13cmholder2 (Autodesk Fusion 360 design; units mm, degrees)
Autodesk Fusion 360 part; units mm, degrees
note: some values were not read from the file. Chosen so that the rebuilt part matches the saved one: that a step has no effect; which face or edge a step refers to. Set by a fixed rule: which sketch regions a step uses.
sketch "Sketch1" plane through (0, 0, 0) normal (1, 0, 0) x (0, 1, 0)
  line L0 (13, -20) -> (-13, 20) construction
  line L1 (-13, -20) -> (13, 20) construction
  line L2 (21.7, -15.8) -> (-8.7, -15.8)
  line L3 (21.7, 15.8) -> (25.9, 15.8)
  line L4 (6.5, -15.8) -> (-34.8, -15.8)
  line L5 (8.6, -15.8) -> (50, -15.8)
  line L6 (50, -15.8) -> (50, -24.8)
  line L7 (50, -24.8) -> (0, -24.8)
  line L8 (-31.55, -27.4) -> (-31.55, 4.2)
  line L9 (-35.75, -15.8) -> (-35.75, 4.2)
  line L10 (-31.55, 4.2) -> (-35.75, 4.2)
  line L11 (-23.95, -27.4) -> (-23.95, 4.2)
  line L12 (-19.75, -27.4) -> (-19.75, 4.2)
  line L13 (-19.75, 4.2) -> (-23.95, 4.2)
  line L14 (-34.8, -15.8) -> (-35.75, -15.8)
  line L15 (-34.8, -20) -> (-35.75, -20)
  line L16 (-35, -24.8) -> (-9, -24.8)
  line L17 (-9, -24.8) -> (0, -24.8)
  line L18 (-35.75, -15.8) -> (-35.75, -24.8)
  line L19 (-35, -24.8) -> (-35.75, -24.8)
  line L20 (-19.75, 4.2) -> (-19.75, 36.6079)
  line L21 (0.25, -15.8) -> (0.25, 36.6079)
  line L22 (-19.75, 36.6079) -> (0.25, 36.6079)
  line L23 (-22.9842, 4.2) -> (-17.5458, 4.2)
  line L24 (-17.5458, 4.2) -> (-17.5458, 36.6079)
  line L25 (-22.6003, 36.6079) -> (-22.9842, 4.2)
  line L26 (-17.5458, 36.6079) -> (-22.6003, 36.6079)
  dimension "d49" = 4.2
  dimension "d50" = 7.6
  dimension "d51" = 4.2
  dimension "d59" = 9
  dimension "d81" = 20
  dimension "d82" = 20
  dimension "d84" = 20
  constraint coincident L0 origin
  constraint coincident L1 origin
  constraint horizontal L4
  constraint midpoint L2 L4.start
  constraint perpendicular L8 L10
  constraint perpendicular L12 L13
  constraint perpendicular L9 L14
  constraint parallel L7 L17
  constraint perpendicular L15 L18
  constraint perpendicular L18 L19
  constraint perpendicular L13 L20
  constraint coincident L4 L21.start
  constraint perpendicular L4 L21
  constraint perpendicular L21 L22
  constraint coincident L13 L23.start
  constraint perpendicular L20 L23
  constraint coincident L22 L24.end
  constraint perpendicular L22 L24
  constraint parallel L22 L26
  measures "d49" distance of L9.end L8.end
  measures "d50" distance of L8 L11
  measures "d51" distance of L11 L12
  measures "d59" distance of L5 L7
  measures "d81" distance of L4 L10
  measures "d82" distance of L4 L13
  measures "d84" distance of L20 L21
extrude "Extrude1" add sketch "Sketch1" along normal mid plane 90 contours L2 L4 L5 L6 L7 L12 L16 L17 | L4 L11 L12 L16 | L4 L8 L11 L16 | L4 L8 L14 L16 L18 L19
extrude "Extrude5" [no effect]
extrude "Extrude6" add sketch "Sketch1" along normal mid plane 90 contours L4 L11 L12 L13 L23 | L4 L8 L9 L10 L14
sketch "Sketch6" plane through (0, -35.75, 0) normal (0, -1, 0) x (1, 0, 0)
  line L0 (-45, -24.8) -> (45, -24.8)
  line L1 (45, -24.8) -> (45, 4.2)
  line L2 (45, 4.2) -> (-45, 4.2)
  line L3 (-45, 4.2) -> (-45, -24.8)
  line L4 (0, 4.2) -> (0, -1.8)
  line L5 (0, -1.8) -> (28.1, -1.8)
  circle A0 centre (28.1, -1.8) radius 3
  line L6 (0, -15.8) -> (0, 4.2)
  circle A1 centre (-28.1, -1.8) radius 3
  line L7 (-24.7214, -20.3) -> (-24.7214, -10.3)
  line L8 (-24.7214, -10.3) -> (-23.398, -10.3)
  line L9 (-23.398, -10.3) -> (-23.398, -20.3)
  line L10 (-23.398, -20.3) -> (-24.7214, -20.3)
  line L11 (-21.0788, -20.3) -> (-21.0788, -10.3)
  line L12 (-21.0788, -10.3) -> (-19.7214, -10.3)
  line L13 (-19.7214, -10.3) -> (-14.469, -18.1513)
  line L14 (-14.469, -18.1513) -> (-14.469, -10.3)
  line L15 (-14.469, -10.3) -> (-13.2002, -10.3)
  line L16 (-13.2002, -10.3) -> (-13.2002, -20.3)
  line L17 (-13.2002, -20.3) -> (-14.5576, -20.3)
  line L18 (-14.5576, -20.3) -> (-19.81, -12.4419)
  line L19 (-19.81, -12.4419) -> (-19.81, -20.3)
  line L20 (-19.81, -20.3) -> (-21.0788, -20.3)
  line L21 (-11.4676, -17.6602) -> (-10.2398, -17.4965)
  spline S0 degree 2 poles (-10.2398, -17.4965) (-10.0283, -18.5401) (-9.5201, -19.0005) knots 0 0 0 1 1 1
  spline S1 degree 2 poles (-9.5201, -19.0005) (-9.0119, -19.461) (-8.2821, -19.461) knots 0 0 0 1 1 1
  spline S2 degree 2 poles (-8.2821, -19.461) (-7.4158, -19.461) (-6.8189, -18.8607) knots 0 0 0 1 1 1
  spline S3 degree 2 poles (-6.8189, -18.8607) (-6.222, -18.2604) (-6.222, -17.3737) knots 0 0 0 1 1 1
  spline S4 degree 2 poles (-6.222, -17.3737) (-6.222, -16.5278) (-6.7746, -15.9787) knots 0 0 0 1 1 1
  spline S5 degree 2 poles (-6.7746, -15.9787) (-7.3271, -15.4296) (-8.1797, -15.4296) knots 0 0 0 1 1 1
  spline S6 degree 2 poles (-8.1797, -15.4296) (-8.5276, -15.4296) (-9.0461, -15.566) knots 0 0 0 1 1 1
  line L22 (-9.0461, -15.566) -> (-8.9096, -14.4883)
  spline S7 degree 2 poles (-8.9096, -14.4883) (-8.7868, -14.5019) (-8.7118, -14.5019) knots 0 0 0 1 1 1
  spline S8 degree 2 poles (-8.7118, -14.5019) (-7.9274, -14.5019) (-7.2998, -14.0926) knots 0 0 0 1 1 1
  spline S9 degree 2 poles (-7.2998, -14.0926) (-6.6722, -13.6834) (-6.6722, -12.8307) knots 0 0 0 1 1 1
  spline S10 degree 2 poles (-6.6722, -12.8307) (-6.6722, -12.1554) (-7.1293, -11.712) knots 0 0 0 1 1 1
  spline S11 degree 2 poles (-7.1293, -11.712) (-7.5863, -11.2686) (-8.3094, -11.2686) knots 0 0 0 1 1 1
  spline S12 degree 2 poles (-8.3094, -11.2686) (-9.0256, -11.2686) (-9.5031, -11.7188) knots 0 0 0 1 1 1
  spline S13 degree 2 poles (-9.5031, -11.7188) (-9.9806, -12.169) (-10.117, -13.0694) knots 0 0 0 1 1 1
  line L23 (-10.117, -13.0694) -> (-11.3448, -12.8512)
  spline S14 degree 2 poles (-11.3448, -12.8512) (-11.1197, -11.6165) (-10.3216, -10.9378) knots 0 0 0 1 1 1
  spline S15 degree 2 poles (-10.3216, -10.9378) (-9.5235, -10.2591) (-8.3366, -10.2591) knots 0 0 0 1 1 1
  spline S16 degree 2 poles (-8.3366, -10.2591) (-7.5181, -10.2591) (-6.8291, -10.6104) knots 0 0 0 1 1 1
  spline S17 degree 2 poles (-6.8291, -10.6104) (-6.1402, -10.9617) (-5.7752, -11.5688) knots 0 0 0 1 1 1
  spline S18 degree 2 poles (-5.7752, -11.5688) (-5.4103, -12.1759) (-5.4103, -12.858) knots 0 0 0 1 1 1
  spline S19 degree 2 poles (-5.4103, -12.858) (-5.4103, -13.506) (-5.7582, -14.0381) knots 0 0 0 1 1 1
  spline S20 degree 2 poles (-5.7582, -14.0381) (-6.1061, -14.5701) (-6.7882, -14.8839) knots 0 0 0 1 1 1
  spline S21 degree 2 poles (-6.7882, -14.8839) (-5.9014, -15.0885) (-5.4103, -15.7332) knots 0 0 0 1 1 1
  spline S22 degree 2 poles (-5.4103, -15.7332) (-4.9192, -16.3778) (-4.9192, -17.3464) knots 0 0 0 1 1 1
  spline S23 degree 2 poles (-4.9192, -17.3464) (-4.9192, -18.6561) (-5.8742, -19.5667) knots 0 0 0 1 1 1
  spline S24 degree 2 poles (-5.8742, -19.5667) (-6.8291, -20.4774) (-8.2889, -20.4774) knots 0 0 0 1 1 1
  spline S25 degree 2 poles (-8.2889, -20.4774) (-9.6054, -20.4774) (-10.4751, -19.6929) knots 0 0 0 1 1 1
  spline S26 degree 2 poles (-10.4751, -19.6929) (-11.3448, -18.9085) (-11.4676, -17.6602) knots 0 0 0 1 1 1
  line L24 (-4.3053, -20.3) -> (-0.4649, -10.3)
  line L25 (-0.4649, -10.3) -> (0.9608, -10.3)
  line L26 (0.9608, -10.3) -> (5.0535, -20.3)
  line L27 (5.0535, -20.3) -> (3.546, -20.3)
  line L28 (3.546, -20.3) -> (2.3796, -17.2714)
  line L29 (2.3796, -17.2714) -> (-1.8018, -17.2714)
  line L30 (-1.8018, -17.2714) -> (-2.9001, -20.3)
  line L31 (-2.9001, -20.3) -> (-4.3053, -20.3)
  line L32 (-1.4199, -16.1936) -> (1.9703, -16.1936)
  line L33 (1.9703, -16.1936) -> (0.9267, -13.4241)
  spline S27 degree 2 poles (0.9267, -13.4241) (0.4492, -12.1622) (0.2173, -11.3505) knots 0 0 0 1 1 1
  spline S28 degree 2 poles (0.2173, -11.3505) (0.0263, -12.3123) (-0.3216, -13.2604) knots 0 0 0 1 1 1
  line L34 (-0.3216, -13.2604) -> (-1.4199, -16.1936)
  spline S29 degree 2 poles (13.6893, -19.2291) (14.6102, -19.8634) (15.3878, -20.1568) knots 0 0 0 1 1 1
  line L35 (15.3878, -20.1568) -> (14.999, -21.0776)
  spline S30 degree 2 poles (14.999, -21.0776) (13.9212, -20.6888) (12.8503, -19.8498) knots 0 0 0 1 1 1
  spline S31 degree 2 poles (12.8503, -19.8498) (11.7384, -20.4705) (10.3946, -20.4705) knots 0 0 0 1 1 1
  spline S32 degree 2 poles (10.3946, -20.4705) (9.0372, -20.4705) (7.9321, -19.8157) knots 0 0 0 1 1 1
  spline S33 degree 2 poles (7.9321, -19.8157) (6.8271, -19.1608) (6.2302, -17.9739) knots 0 0 0 1 1 1
  spline S34 degree 2 poles (6.2302, -17.9739) (5.6333, -16.787) (5.6333, -15.3) knots 0 0 0 1 1 1
  spline S35 degree 2 poles (5.6333, -15.3) (5.6333, -13.8198) (6.2336, -12.6056) knots 0 0 0 1 1 1
  spline S36 degree 2 poles (6.2336, -12.6056) (6.8339, -11.3914) (7.9424, -10.757) knots 0 0 0 1 1 1
  spline S37 degree 2 poles (7.9424, -10.757) (9.0508, -10.1226) (10.4219, -10.1226) knots 0 0 0 1 1 1
  spline S38 degree 2 poles (10.4219, -10.1226) (11.8066, -10.1226) (12.9185, -10.7809) knots 0 0 0 1 1 1
  spline S39 degree 2 poles (12.9185, -10.7809) (14.0303, -11.4392) (14.6136, -12.6226) knots 0 0 0 1 1 1
  spline S40 degree 2 poles (14.6136, -12.6226) (15.1968, -13.8061) (15.1968, -15.2932) knots 0 0 0 1 1 1
  spline S41 degree 2 poles (15.1968, -15.2932) (15.1968, -16.5278) (14.8216, -17.5135) knots 0 0 0 1 1 1
  spline S42 degree 2 poles (14.8216, -17.5135) (14.4464, -18.4992) (13.6893, -19.2291) knots 0 0 0 1 1 1
  spline S43 degree 2 poles (10.7766, -17.5374) (11.9226, -17.858) (12.6661, -18.4924) knots 0 0 0 1 1 1
  spline S44 degree 2 poles (12.6661, -18.4924) (13.8325, -17.4282) (13.8325, -15.2932) knots 0 0 0 1 1 1
  spline S45 degree 2 poles (13.8325, -15.2932) (13.8325, -14.079) (13.4198, -13.1718) knots 0 0 0 1 1 1
  spline S46 degree 2 poles (13.4198, -13.1718) (13.0072, -12.2645) (12.2125, -11.7632) knots 0 0 0 1 1 1
  spline S47 degree 2 poles (12.2125, -11.7632) (11.4178, -11.2618) (10.4287, -11.2618) knots 0 0 0 1 1 1
  spline S48 degree 2 poles (10.4287, -11.2618) (8.9485, -11.2618) (7.973, -12.2748) knots 0 0 0 1 1 1
  spline S49 degree 2 poles (7.973, -12.2748) (6.9976, -13.2877) (6.9976, -15.3) knots 0 0 0 1 1 1
  spline S50 degree 2 poles (6.9976, -15.3) (6.9976, -17.2509) (7.9628, -18.2945) knots 0 0 0 1 1 1
  spline S51 degree 2 poles (7.9628, -18.2945) (8.928, -19.3382) (10.4287, -19.3382) knots 0 0 0 1 1 1
  spline S52 degree 2 poles (10.4287, -19.3382) (11.1381, -19.3382) (11.7657, -19.0722) knots 0 0 0 1 1 1
  spline S53 degree 2 poles (11.7657, -19.0722) (11.1449, -18.6697) (10.456, -18.4992) knots 0 0 0 1 1 1
  line L36 (10.456, -18.4992) -> (10.7766, -17.5374)
  line L37 (16.9226, -20.3) -> (16.9226, -10.3)
  line L38 (16.9226, -10.3) -> (18.2459, -10.3)
  line L39 (18.2459, -10.3) -> (18.2459, -15.2591)
  line L40 (18.2459, -15.2591) -> (23.2118, -10.3)
  line L41 (23.2118, -10.3) -> (25.0058, -10.3)
  line L42 (25.0058, -10.3) -> (20.8107, -14.3518)
  line L43 (20.8107, -14.3518) -> (25.19, -20.3)
  line L44 (25.19, -20.3) -> (23.4437, -20.3)
  line L45 (23.4437, -20.3) -> (19.883, -15.2386)
  line L46 (19.883, -15.2386) -> (18.2459, -16.8348)
  line L47 (18.2459, -16.8348) -> (18.2459, -20.3)
  line L48 (18.2459, -20.3) -> (16.9226, -20.3)
  dimension "d54" = 6
  dimension "d55" = 28.1
  dimension "d56" = 6
  constraint midpoint L2 L4.start
  constraint perpendicular L2 L4
  constraint perpendicular L4 L5
  constraint coincident L5.end A0.centre
  constraint symmetric A0 L6 A1
  measures "d54" distance of L4.start L4.end
  measures "d55" distance of L4.end L5.end
  measures "d56" diameter of A0
extrude "Extrude11" cut sketch "Sketch6" against normal blind 2 contours L7 L8 L9 L10 | L11 L12 L13 L14 L15 L16 L17 L18 L19 L20 | L21 S0 S1 S2 S3 S4 S5 S6 L22 S7 S8 S9 S10 S11 S12 S13 L23 S14 S15 S16 S17 S18 S19 S20 S21 S22 S23 S24 S25 S26 | L24 L25 L26 L27 L28 L29 L30 L31 | S29 L35 S30 S31 S32 S33 S34 S35 S36 S37 S38 S39 S40 S41 S42 | L37 L38 L39 L40 L41 L42 L43 L44 L45 L46 L47 L48
extrude "Extrude7" cut sketch "Sketch6" against normal blind 23 contours A0 | A1
sketch "Sketch7" plane through (0, 0, -24.8) normal (0, 0, -1) x (1, 0, 0)
  line L0 (-45, -50) -> (45, -50)
  line L1 (45, -50) -> (45, 35.75)
  line L2 (45, 35.75) -> (-45, 35.75)
  line L3 (-45, 35.75) -> (-45, -50)
  circle A0 centre (0, 4.875) radius 4.65
  dimension "d61" = 9.3
  measures "d61" diameter of A0
extrude "Extrude8" cut sketch "Sketch7" against normal blind 8 contours A0
sketch "Sketch8" plane through (0, 0, 0) normal (0, 0, 1) x (1, 0, 0)
  line L0 (-45, 50) -> (-45, -19.75)
  line L1 (45, -19.75) -> (45, 50)
  line L2 (45, 50) -> (-45, 50)
  line L3 (0, 8.6) -> (0, 50)
  line L4 (-40, 50) -> (-45, 50)
  line L5 (-45, 43.0231) -> (-45, 50)
  line L6 (-45, 50) -> (-45, -19.75)
  line L7 (-40, 50) -> (-40, -19.75)
  line L8 (-44, -19.75) -> (-45, -19.75)
  line L9 (-45, -19.75) -> (-40, -19.75)
  line L10 (-13.8, 50) -> (-13.8, -20)
  line L11 (-8.8, 50) -> (-8.8, -19.75)
  line L12 (-13.8, 50) -> (-8.8, 50)
  line L13 (-13.8, -20) -> (-8.8, -19.75)
  line L14 (-45, -19.75) -> (45, -19.75)
  dimension "d76" = 5
  dimension "d77" = 26.2
  dimension "d78" = 5
  dimension "d83" = 69.75
  constraint coincident L0 L5.start
  constraint perpendicular L4 L5
  constraint perpendicular L4 L6
  constraint coincident L2 L4.start
  constraint coincident L0 L6.end
  constraint coincident L2 L10.start
  constraint perpendicular L2 L10
  constraint coincident L2 L11.start
  measures "d76" distance of L6 L7
  measures "d77" distance of L7 L10
  measures "d78" distance of L10 L11
  measures "d83" distance of L4 L9
extrude "Extrude9" add sketch "Sketch8" along normal mid plane 48 contours L0 L2 L4 L5 L6 L7 L8 L9 L14 | L2 L10 L11 L12 L14 | L10 L13 L14
extrude "Extrude10" cut sketch "Sketch1" along normal mid plane 170 contours L2 L4 L12 L21 L22 L23 L24 | L20 L22 L23 L24 L26
extrude "Extrude12" cut sketch "Sketch1" along normal mid plane 38 contours L2 L4 L12 L21 L22 L23 L24 | L20 L22 L23 L24 L26 | L13 L20 L23 L25 L26
fillet "Fillet16" radius 1 17 edges at (-45, -35.75, -10.3) (45, -35.75, -10.3) (45, -31.55, -5.8) (-45, -31.55, -5.8) (-45, -23.95, -5.8) (-45, -19.75, -5.8) (45, -19.75, -5.8) (45, -23.95, -5.8) (-45, 50, -0.4) (-40, 50, 4.1) (-13.8, 50, 4.1) (-8.8, 50, 4.1) (45, 50, -20.3) (-45, 0.25, 4.1) (-40, 0.25, 4.1) (-13.8, 0.25, 4.1) (-8.8, 0.25, 4.1)
